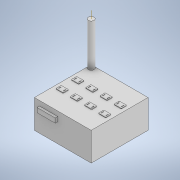
# Autodesk Inventor part: Prototipo
Saved by Autodesk Inventor 2022 (Build 260153000, 153)
## iProperties
Created: 2022-03-12
Part Number: Prototipo
Material: Genérico
Document SubType Name: Modeling
Designer: jlara
Density: 1 g/cm^3
Appearance: Valor por defecto
Author: jlara
Autodesk Inventor part; units mm, degrees
ref_plane "YZ Plane" through (0, 0, 0) normal (1, 0, 0) x (0, 1, 0)
ref_plane "XZ Plane" through (0, 0, 0) normal (0, 1, 0) x (-1, 0, 0)
ref_plane "XY Plane" through (0, 0, 0) normal (0, 0, 1) x (1, 0, 0)
sketch "Boceto1" plane through (0, 0, 0) normal (0, 1, 0) x (-1, 0, 0)
  line L0 (-100, 100) -> (100, 100)
  line L1 (100, 100) -> (100, -100)
  line L2 (100, -100) -> (-100, -100)
  line L3 (-100, -100) -> (-100, 100)
  line L4 (-100, 100) -> (100, -100) construction
  line L5 (100, 100) -> (-100, -100) construction
  point P0 (0, 0)
  dimension "d0" = 200
  dimension "d3" = 200
  constraints: 12 end point, 2 midpoint, 2 parallel, 1 horizontal, 1 perpendicular
  measures "d0" distance of L0.start L0.end
  measures "d3" distance of L2.end L0.start
extrude "Extrusión1" add sketch "Boceto1" along normal blind 100
sketch "Boceto2" plane through (0, 100, 0) normal (0, 1, 0) x (1, 0, 0)
  line L0 (-100, 100) -> (-100, -100) projected
  line L1 (-100, 80) -> (0, 80) construction
  line L2 (100, 100) -> (-100, 100) construction
  line L3 (-100, 100) -> (0, 100) construction
  circle A0 centre (-90, 90) radius 10
  point P0 (0, 0)
  dimension "d4" = 20
  constraints: 4 end point, 3 tangent, 1 centre point, 1 midpoint, 1 perpendicular, 1 point on line
  measures "d4" distance of L0.start L1.start
extrude "Extrusión2" add sketch "Boceto2" along normal blind 150
sketch "Boceto3" plane through (0, 100, 0) normal (0, 1, 0) x (1, 0, 0)
  line L0 (0, 0) -> (0, 54.6157) construction
  line L1 (0, 54.6157) -> (-100, 54.6157) construction
  line L2 (-100, 100) -> (-100, -100) projected
  line L3 (-50, 54.6157) -> (-50, 0) construction
  line L4 (100, -100) -> (100, 100) projected
  line L5 (0, 54.6157) -> (100, 54.6157) construction
  line L6 (50, 54.6157) -> (50, 0) construction
  line L7 (-100, 0) -> (100, 0) construction
  line L8 (0, -54.6157) -> (-100, -54.6157) construction
  line L9 (-50, -54.6157) -> (-50, 0) construction
  line L10 (0, -54.6157) -> (100, -54.6157) construction
  line L11 (50, -54.6157) -> (50, 0) construction
  line L12 (-75, 27.3078) -> (-75, 54.6157) construction
  line L13 (-86, 36.8328) -> (-64, 36.8328)
  line L14 (-62, 34.8328) -> (-62, 19.7828)
  line L15 (-64, 17.7828) -> (-86, 17.7828)
  line L16 (-88, 19.7828) -> (-88, 34.8328)
  line L17 (-88, 36.8328) -> (-62, 17.7828) construction
  line L18 (-62, 36.8328) -> (-88, 17.7828) construction
  line L19 (-75, 27.3078) -> (-83.255, 27.3078) construction
  line L20 (-83.255, 27.3078) -> (-83.255, 31.4328) construction
  line L21 (-84.005, 23.1828) -> (-82.505, 23.1828)
  line L22 (-82.505, 23.1828) -> (-82.505, 31.4328)
  line L23 (-82.505, 31.4328) -> (-84.005, 31.4328)
  line L24 (-84.005, 31.4328) -> (-84.005, 23.1828)
  line L25 (-84.005, 23.1828) -> (-82.505, 31.4328) construction
  line L26 (-82.505, 23.1828) -> (-84.005, 31.4328) construction
  line L27 (-66.745, 27.3078) -> (-66.745, 31.4328) construction
  line L28 (-65.995, 23.1828) -> (-67.495, 23.1828)
  line L29 (-67.495, 23.1828) -> (-67.495, 31.4328)
  line L30 (-67.495, 31.4328) -> (-65.995, 31.4328)
  line L31 (-65.995, 31.4328) -> (-65.995, 23.1828)
  line L32 (-65.995, 23.1828) -> (-67.495, 31.4328) construction
  line L33 (-67.495, 23.1828) -> (-65.995, 31.4328) construction
  arc A0 (-86, 36.8328) -> (-88, 34.8328) centre (-86, 34.8328) ccw
  arc A1 (-62, 34.8328) -> (-64, 36.8328) centre (-64, 34.8328) ccw
  arc A2 (-88, 19.7828) -> (-86, 17.7828) centre (-86, 19.7828) ccw
  arc A3 (-64, 17.7828) -> (-62, 19.7828) centre (-64, 19.7828) ccw
  line L34 (-25, 27.3078) -> (-25, 54.6157) construction
  line L35 (-14, 36.8328) -> (-36, 36.8328)
  line L36 (-38, 34.8328) -> (-38, 19.7828)
  line L37 (-36, 17.7828) -> (-14, 17.7828)
  line L38 (-12, 19.7828) -> (-12, 34.8328)
  line L39 (-12, 36.8328) -> (-38, 17.7828) construction
  line L40 (-38, 36.8328) -> (-12, 17.7828) construction
  line L41 (-25, 27.3078) -> (-16.745, 27.3078) construction
  line L42 (-16.745, 27.3078) -> (-16.745, 31.4328) construction
  line L43 (-15.995, 23.1828) -> (-17.495, 23.1828)
  line L44 (-17.495, 23.1828) -> (-17.495, 31.4328)
  line L45 (-17.495, 31.4328) -> (-15.995, 31.4328)
  line L46 (-15.995, 31.4328) -> (-15.995, 23.1828)
  line L47 (-15.995, 23.1828) -> (-17.495, 31.4328) construction
  line L48 (-17.495, 23.1828) -> (-15.995, 31.4328) construction
  line L49 (-34.005, 23.1828) -> (-32.505, 23.1828)
  line L50 (-32.505, 23.1828) -> (-32.505, 31.4328)
  line L51 (-34.005, 31.4328) -> (-34.005, 23.1828)
  line L52 (-34.005, 23.1828) -> (-32.505, 31.4328) construction
  line L53 (-32.505, 23.1828) -> (-34.005, 31.4328) construction
  line L54 (-33.255, 27.3078) -> (-33.255, 31.4328) construction
  line L55 (-32.505, 31.4328) -> (-34.005, 31.4328)
  arc A4 (-12, 34.8328) -> (-14, 36.8328) centre (-14, 34.8328) ccw
  arc A5 (-36, 36.8328) -> (-38, 34.8328) centre (-36, 34.8328) ccw
  arc A6 (-14, 17.7828) -> (-12, 19.7828) centre (-14, 19.7828) ccw
  arc A7 (-38, 19.7828) -> (-36, 17.7828) centre (-36, 19.7828) ccw
  line L56 (86, 36.8328) -> (64, 36.8328)
  line L57 (62, 34.8328) -> (62, 19.7828)
  line L58 (64, 17.7828) -> (86, 17.7828)
  line L59 (88, 19.7828) -> (88, 34.8328)
  line L60 (88, 36.8328) -> (62, 17.7828) construction
  line L61 (62, 36.8328) -> (88, 17.7828) construction
  line L62 (75, 27.3078) -> (83.255, 27.3078) construction
  line L63 (83.255, 27.3078) -> (83.255, 31.4328) construction
  line L64 (84.005, 23.1828) -> (82.505, 23.1828)
  line L65 (82.505, 23.1828) -> (82.505, 31.4328)
  line L66 (82.505, 31.4328) -> (84.005, 31.4328)
  line L67 (84.005, 31.4328) -> (84.005, 23.1828)
  line L68 (84.005, 23.1828) -> (82.505, 31.4328) construction
  line L69 (82.505, 23.1828) -> (84.005, 31.4328) construction
  line L70 (65.995, 23.1828) -> (67.495, 23.1828)
  line L71 (67.495, 23.1828) -> (67.495, 31.4328)
  line L72 (65.995, 31.4328) -> (65.995, 23.1828)
  line L73 (65.995, 23.1828) -> (67.495, 31.4328) construction
  line L74 (67.495, 23.1828) -> (65.995, 31.4328) construction
  line L75 (66.745, 27.3078) -> (66.745, 31.4328) construction
  line L76 (67.495, 31.4328) -> (65.995, 31.4328)
  arc A8 (88, 34.8328) -> (86, 36.8328) centre (86, 34.8328) ccw
  arc A9 (64, 36.8328) -> (62, 34.8328) centre (64, 34.8328) ccw
  arc A10 (86, 17.7828) -> (88, 19.7828) centre (86, 19.7828) ccw
  arc A11 (62, 19.7828) -> (64, 17.7828) centre (64, 19.7828) ccw
  arc A12 (36, 17.7828) -> (38, 19.7828) centre (36, 19.7828) ccw
  line L77 (34.005, 23.1828) -> (32.505, 23.1828)
  line L78 (32.505, 23.1828) -> (32.505, 31.4328)
  line L79 (34.005, 23.1828) -> (32.505, 31.4328) construction
  line L80 (32.505, 23.1828) -> (34.005, 31.4328) construction
  line L81 (32.505, 31.4328) -> (34.005, 31.4328)
  line L82 (34.005, 31.4328) -> (34.005, 23.1828)
  line L83 (38, 34.8328) -> (38, 19.7828)
  arc A13 (38, 34.8328) -> (36, 36.8328) centre (36, 34.8328) ccw
  line L84 (33.255, 27.3078) -> (33.255, 31.4328) construction
  line L85 (14, 36.8328) -> (36, 36.8328)
  line L86 (36, 17.7828) -> (14, 17.7828)
  line L87 (12, 19.7828) -> (12, 34.8328)
  line L88 (12, 36.8328) -> (38, 17.7828) construction
  line L89 (38, 36.8328) -> (12, 17.7828) construction
  line L90 (25, 27.3078) -> (16.745, 27.3078) construction
  line L91 (16.745, 27.3078) -> (16.745, 31.4328) construction
  line L92 (15.995, 23.1828) -> (17.495, 23.1828)
  line L93 (17.495, 23.1828) -> (17.495, 31.4328)
  line L94 (15.995, 31.4328) -> (15.995, 23.1828)
  line L95 (15.995, 23.1828) -> (17.495, 31.4328) construction
  line L96 (17.495, 23.1828) -> (15.995, 31.4328) construction
  arc A14 (12, 19.7828) -> (14, 17.7828) centre (14, 19.7828) ccw
  arc A15 (14, 36.8328) -> (12, 34.8328) centre (14, 34.8328) ccw
  line L97 (17.495, 31.4328) -> (15.995, 31.4328)
  line L98 (-86, -36.8328) -> (-64, -36.8328)
  line L99 (-62, -34.8328) -> (-62, -19.7828)
  line L100 (-64, -17.7828) -> (-86, -17.7828)
  line L101 (-88, -19.7828) -> (-88, -34.8328)
  line L102 (-88, -36.8328) -> (-62, -17.7828) construction
  line L103 (-62, -36.8328) -> (-88, -17.7828) construction
  line L104 (-75, -27.3078) -> (-83.255, -27.3078) construction
  line L105 (-83.255, -27.3078) -> (-83.255, -31.4328) construction
  line L106 (-84.005, -23.1828) -> (-82.505, -23.1828)
  line L107 (-82.505, -23.1828) -> (-82.505, -31.4328)
  line L108 (-82.505, -31.4328) -> (-84.005, -31.4328)
  line L109 (-84.005, -31.4328) -> (-84.005, -23.1828)
  line L110 (-84.005, -23.1828) -> (-82.505, -31.4328) construction
  line L111 (-82.505, -23.1828) -> (-84.005, -31.4328) construction
  line L112 (-65.995, -23.1828) -> (-67.495, -23.1828)
  line L113 (-67.495, -23.1828) -> (-67.495, -31.4328)
  line L114 (-65.995, -31.4328) -> (-65.995, -23.1828)
  line L115 (-65.995, -23.1828) -> (-67.495, -31.4328) construction
  line L116 (-67.495, -23.1828) -> (-65.995, -31.4328) construction
  line L117 (-66.745, -27.3078) -> (-66.745, -31.4328) construction
  line L118 (-67.495, -31.4328) -> (-65.995, -31.4328)
  arc A16 (-88, -34.8328) -> (-86, -36.8328) centre (-86, -34.8328) ccw
  arc A17 (-64, -36.8328) -> (-62, -34.8328) centre (-64, -34.8328) ccw
  arc A18 (-86, -17.7828) -> (-88, -19.7828) centre (-86, -19.7828) ccw
  arc A19 (-62, -19.7828) -> (-64, -17.7828) centre (-64, -19.7828) ccw
  arc A20 (-36, -17.7828) -> (-38, -19.7828) centre (-36, -19.7828) ccw
  line L119 (-34.005, -23.1828) -> (-32.505, -23.1828)
  line L120 (-32.505, -23.1828) -> (-32.505, -31.4328)
  line L121 (-34.005, -23.1828) -> (-32.505, -31.4328) construction
  line L122 (-32.505, -23.1828) -> (-34.005, -31.4328) construction
  line L123 (-32.505, -31.4328) -> (-34.005, -31.4328)
  line L124 (-34.005, -31.4328) -> (-34.005, -23.1828)
  line L125 (-38, -34.8328) -> (-38, -19.7828)
  arc A21 (-38, -34.8328) -> (-36, -36.8328) centre (-36, -34.8328) ccw
  line L126 (-33.255, -27.3078) -> (-33.255, -31.4328) construction
  line L127 (-14, -36.8328) -> (-36, -36.8328)
  line L128 (-36, -17.7828) -> (-14, -17.7828)
  line L129 (-12, -19.7828) -> (-12, -34.8328)
  line L130 (-12, -36.8328) -> (-38, -17.7828) construction
  line L131 (-38, -36.8328) -> (-12, -17.7828) construction
  line L132 (-25, -27.3078) -> (-16.745, -27.3078) construction
  line L133 (-16.745, -27.3078) -> (-16.745, -31.4328) construction
  line L134 (-15.995, -23.1828) -> (-17.495, -23.1828)
  line L135 (-17.495, -23.1828) -> (-17.495, -31.4328)
  line L136 (-15.995, -31.4328) -> (-15.995, -23.1828)
  line L137 (-15.995, -23.1828) -> (-17.495, -31.4328) construction
  line L138 (-17.495, -23.1828) -> (-15.995, -31.4328) construction
  arc A22 (-12, -19.7828) -> (-14, -17.7828) centre (-14, -19.7828) ccw
  arc A23 (-14, -36.8328) -> (-12, -34.8328) centre (-14, -34.8328) ccw
  line L139 (-17.495, -31.4328) -> (-15.995, -31.4328)
  line L140 (62, -34.8328) -> (62, -19.7828)
  line L141 (64, -17.7828) -> (86, -17.7828)
  line L142 (88, -36.8328) -> (62, -17.7828) construction
  line L143 (62, -36.8328) -> (88, -17.7828) construction
  line L144 (86, -36.8328) -> (64, -36.8328)
  line L145 (75, -27.3078) -> (83.255, -27.3078) construction
  line L146 (82.505, -23.1828) -> (82.505, -31.4328)
  arc A24 (88, -19.7828) -> (86, -17.7828) centre (86, -19.7828) ccw
  line L147 (83.255, -27.3078) -> (83.255, -31.4328) construction
  line L148 (84.005, -23.1828) -> (82.505, -31.4328) construction
  line L149 (82.505, -23.1828) -> (84.005, -31.4328) construction
  line L150 (84.005, -31.4328) -> (84.005, -23.1828)
  line L151 (82.505, -31.4328) -> (84.005, -31.4328)
  line L152 (88, -19.7828) -> (88, -34.8328)
  arc A25 (86, -36.8328) -> (88, -34.8328) centre (86, -34.8328) ccw
  line L153 (84.005, -23.1828) -> (82.505, -23.1828)
  line L154 (67.495, -31.4328) -> (65.995, -31.4328)
  line L155 (66.745, -27.3078) -> (66.745, -31.4328) construction
  line L156 (67.495, -23.1828) -> (67.495, -31.4328)
  arc A26 (62, -34.8328) -> (64, -36.8328) centre (64, -34.8328) ccw
  line L157 (65.995, -23.1828) -> (67.495, -23.1828)
  line L158 (65.995, -23.1828) -> (67.495, -31.4328) construction
  line L159 (67.495, -23.1828) -> (65.995, -31.4328) construction
  line L160 (65.995, -31.4328) -> (65.995, -23.1828)
  arc A27 (64, -17.7828) -> (62, -19.7828) centre (64, -19.7828) ccw
  arc A28 (38, -19.7828) -> (36, -17.7828) centre (36, -19.7828) ccw
  line L161 (38, -34.8328) -> (38, -19.7828)
  arc A29 (36, -36.8328) -> (38, -34.8328) centre (36, -34.8328) ccw
  line L162 (34.005, -31.4328) -> (34.005, -23.1828)
  line L163 (34.005, -23.1828) -> (32.505, -23.1828)
  line L164 (33.255, -27.3078) -> (33.255, -31.4328) construction
  line L165 (32.505, -31.4328) -> (34.005, -31.4328)
  line L166 (32.505, -23.1828) -> (32.505, -31.4328)
  line L167 (34.005, -23.1828) -> (32.505, -31.4328) construction
  line L168 (32.505, -23.1828) -> (34.005, -31.4328) construction
  line L169 (25, -27.3078) -> (16.745, -27.3078) construction
  line L170 (36, -17.7828) -> (14, -17.7828)
  line L171 (12, -36.8328) -> (38, -17.7828) construction
  line L172 (38, -36.8328) -> (12, -17.7828) construction
  line L173 (12, -19.7828) -> (12, -34.8328)
  line L174 (14, -36.8328) -> (36, -36.8328)
  arc A30 (12, -34.8328) -> (14, -36.8328) centre (14, -34.8328) ccw
  line L175 (17.495, -31.4328) -> (15.995, -31.4328)
  line L176 (16.745, -27.3078) -> (16.745, -31.4328) construction
  line L177 (15.995, -31.4328) -> (15.995, -23.1828)
  line L178 (17.495, -23.1828) -> (17.495, -31.4328)
  line L179 (15.995, -23.1828) -> (17.495, -23.1828)
  line L180 (17.495, -23.1828) -> (15.995, -31.4328) construction
  line L181 (15.995, -23.1828) -> (17.495, -31.4328) construction
  arc A31 (14, -17.7828) -> (12, -19.7828) centre (14, -19.7828) ccw
  dimension "d18" = 26
  dimension "d19" = 19.05
  dimension "d20" = 8.255
  dimension "d22" = 4.125
  dimension "d23" = 1.5
  dimension "d24" = 2
  constraints: 360 end point, 227 symmetric about line, 64 point on circle, 51 midpoint, 32 centre point, 18 point on line, 4 horizontal, 4 parallel, 3 perpendicular, 3 vertical, 2 tangent, 31 other
  measures "d18" distance of L17.end L18.end
  measures "d19" distance of L18.start L17.end
  measures "d20" distance of L12.start L19.end
  measures "d22" distance of L19.end L20.end
  measures "d23" distance of L23.end L22.end
  measures "d24" radius of A0
extrude "Extrusión3" add sketch "Boceto3" along normal blind 2
sketch "Boceto4" plane through (-100, 0, 100) normal (0, 0, 1) x (1, 0, 0)
  line L0 (100, 0) -> (100, 100) construction
  line L1 (0, 100) -> (200, 100) construction
  line L2 (0, 0) -> (0, 100) construction
  line L3 (200, 0) -> (200, 100) projected
  line L4 (200, 50) -> (0, 50) construction
  line L5 (0, 100) -> (0, 50) construction
  line L6 (0, 100) -> (100, 100) construction
  line L7 (50, 100) -> (50, 50) construction
  line L8 (50, 75) -> (0, 75) construction
  line L9 (50, 75) -> (100, 75) construction
  line L10 (17.75, 67) -> (82.25, 67)
  line L11 (82.25, 67) -> (82.25, 83)
  line L12 (82.25, 83) -> (17.75, 83)
  line L13 (17.75, 83) -> (17.75, 67)
  line L14 (17.75, 67) -> (82.25, 83) construction
  line L15 (82.25, 67) -> (17.75, 83) construction
  dimension "d27" = 64.5
  dimension "d28" = 16
  constraints: 26 end point, 8 midpoint, 2 horizontal, 2 parallel, 2 perpendicular, 1 point on line, 1 symmetric about line, 1 vertical
  measures "d27" distance of L12.end L11.end
  measures "d28" distance of L11.end L10.end
extrude "Extrusión4" add sketch "Boceto4" along normal blind 8.5
